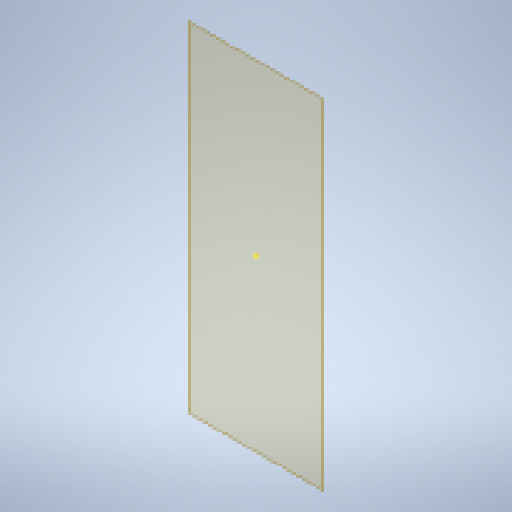
# Autodesk Inventor part: SmallBeltClampCover
Saved by Autodesk Inventor 2023 (Build 270158000, 158)
## iProperties
Created: 2023-09-08
Part Number: SmallBeltClampCover
Material: Generic
Document SubType Name: Modeling
Designer: Felix
Density: 1 g/cm^3
Appearance: Default
Author: Felix
Autodesk Inventor part; units mm, degrees
ref_plane "YZ Plane" through (0, 0, 0) normal (1, 0, 0) x (0, 1, 0)
ref_plane "XZ Plane" through (0, 0, 0) normal (0, 1, 0) x (-1, 0, 0)
ref_plane "XY Plane" through (0, 0, 0) normal (0, 0, 1) x (1, 0, 0)
ref_plane "Work Plane2" through (-0.0047, 0, -9.2) normal (-0.001, 0, -1) x (-1, 0, 0.001)
sketch "Sketch2" plane through (-0.0047, 0, -9.2) normal (-0.001, 0, -1) x (-1, 0, 0.001)
  line L0 (6, 2.0218) -> (3.5, 15.0218) projected
  line L1 (6, -1.9782) -> (6, 2.0218) projected
  line L2 (2.5, -15.0218) -> (6, -1.9782) projected
  line L3 (3.5, 15.0218) -> (-3.5, 15.0218) projected
  line L4 (-3.5, 15.0218) -> (-6, 2.0218) projected
  line L5 (-6, 2.0218) -> (-6, -1.9782) projected
  line L6 (-6, -1.9782) -> (-2.5, -15.0218) projected
  line L7 (1.25, -15.0218) -> (2.5, -15.0218) projected
  line L8 (-2.5, -15.0218) -> (-1.25, -15.0218) projected
  line L9 (1.25, -15.0218) -> (-1.25, -15.0218)
  circle A0 centre (0, 0.0218) radius 1.7 projected
  point P0 (0.0047, 0)
  constraints: 2 end point, 1 horizontal
extrude "Extrusion1" add sketch "Sketch2" along normal blind 2
sketch "Sketch3" plane through (-0.0047, 0, -9.2) normal (0.001, 0, 1) x (1, 0, -0.001)
  line L0 (1.25, -15.0218) -> (1.25, -5.0218) construction
  line L1 (-1.25, -5.0218) -> (-1.25, -15.0218) construction
  line L2 (2.5, -15.0218) -> (-2.5, -15.0218) projected
  line L3 (1.05, -5.2218) -> (-1.05, -5.2218)
  line L4 (-1.05, -5.2218) -> (-1.05, -15.0218)
  line L5 (-1.05, -15.0218) -> (1.05, -15.0218)
  line L6 (1.05, -15.0218) -> (1.05, -5.2218)
  point P0 (-0.0047, 0)
  point P1 (1.05, -15.0218)
  dimension "d2" = 0.2
  dimension "d3" = 0.2
  dimension "d4" = 0.2
  constraints: 8 end point, 2 parallel, 1 horizontal, 1 perpendicular, 1 point on line
  measures "d2" distance between parallel lines of L0 L6
  measures "d3" distance between parallel lines of L1 L4
  measures "d4" distance from line of L0.end L3
extrude "Extrusion2" add sketch "Sketch3" along normal blind 1
equation "\"d3\" = d2"
equation "\"d4\" = d2"
body "Solid1"
